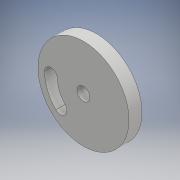
# Autodesk Inventor part: Part6-01
Saved by Autodesk Inventor 2017 (Build 210142000, 142)
## iProperties
Created: 2021-05-19
Part Number: Part6-01
Material: Generic
Document SubType Name: Modeling
Designer: majch
Density: 1 g/cm^3
Appearance: Default
Author: majch
Autodesk Inventor part; units mm, degrees
ref_plane "YZ Plane" through (0, 0, 0) normal (1, 0, 0) x (0, 1, 0)
ref_plane "XZ Plane" through (0, 0, 0) normal (0, 1, 0) x (-1, 0, 0)
ref_plane "XY Plane" through (0, 0, 0) normal (0, 0, 1) x (1, 0, 0)
sketch "Sketch1" plane through (0, 0, 0) normal (0, 1, 0) x (-1, 0, 0)
  circle A0 centre (0, 0) radius 17.5
  dimension "d0" = 35
  constraints: 1 centre point, 1 coincident
  measures "d0" diameter of A0
extrude "Extrusion1" add sketch "Sketch1" along normal blind 5
sketch "Sketch2" plane through (0, 5, 0) normal (0, 1, 0) x (1, 0, 0)
  arc A0 (-10.6066, 10.6066) -> (-15, 0) centre (0, 0) ccw
  line L0 (0, 0) -> (-10.6066, 10.6066) construction
  line L1 (0, 0) -> (-15, 0) construction
  arc A1 (-7.0711, 7.0711) -> (-10, 0) centre (0, 0) ccw
  arc A2 (-15, 0) -> (-10, 0) centre (-12.5, 0) ccw
  arc A3 (-7.0711, 7.0711) -> (-10.6066, 10.6066) centre (-8.8388, 8.8388) ccw
  dimension "kat" = 45
  dimension "d8" = 45
  constraints: 8 point on circle, 4 centre point, 4 end point, 3 point on line, 1 coincident
extrude "Extrusion2" cut sketch "Sketch2" against normal through all
sketch "Sketch3" plane through (0, 5, 0) normal (0, 1, 0) x (1, 0, 0)
  circle A0 centre (0, 0) radius 2.5
  dimension "d11" = 5
  constraints: 1 centre point, 1 coincident
  measures "d11" diameter of A0
extrude "Extrusion3" cut sketch "Sketch3" against normal through all
equation "\"d8\" = kat"
body "Solid1"
